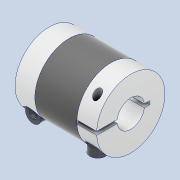
# Autodesk Inventor part: Coupling_SOH-16C-5×6_自作モデル
Saved by Autodesk Inventor 2021.2 (Build 252289000, 289)
## iProperties
Created: 2021-02-28
Part Number: Coupling_SOH-16C-5×6_自作モデル
Material: アルミニウム 6061
Document SubType Name: Modeling
Designer: Hagihara Yuya
Density: 2.7 g/cm^3
Appearance: アルミニウム - フラット
Author: Hagihara Yuya
Autodesk Inventor part; units mm, degrees
sketch "スケッチ1" plane through (0, 0, 0) normal (1, 0, 0) x (0, 1, 0)
  circle A0 centre (0, 0) radius 10
  dimension "d0" = 20
  constraints: 1 centre point, 1 coincident
  measures "d0" diameter of A0
extrude "押し出し1" add sketch "スケッチ1" along normal blind 23.9
sketch "スケッチ2" plane through (23.9, 0, 0) normal (1, 0, 0) x (0, 0, -1)
  point P0 (0, 0)
  point P1 (0, 0)
  constraints: 1 coincident
hole "軸穴1" at (23.9, 0, 0) direction (-1, 0, 0) diameter 8 depth 11
sketch "スケッチ3" plane through (0, 0, 0) normal (-1, 0, 0) x (0, 0, 1)
  point P0 (0, 0)
  point P1 (0, 0)
  constraints: 1 coincident
hole "軸穴2" at (0, 0, 0) direction (1, 0, 0) diameter 8 depth 11
ref_plane "作業平面1" through (5.8, 0, 0) normal (-1, 0, 0) x (0, 0, 1)
sketch "スケッチ4" plane through (5.8, 0, 0) normal (-1, 0, 0) x (0, 0, 1)
  circle A0 centre (0, 0) radius 9.99
  circle A1 centre (0, 0) radius 10 projected
  dimension "d18" = 0.01
  constraints: 1 centre point, 1 coincident
  measures "d18" radial gap between concentric circles of A1 A0
extrude "押し出し2" cut sketch "スケッチ4" against normal blind 12.3
sketch "スケッチ5" plane through (23.9, 0, 0) normal (1, 0, 0) x (0, 0, -1)
  line L0 (-5.5, -0.5) -> (10, -0.5)
  line L1 (10, -0.5) -> (10, 0.5)
  line L2 (10, 0.5) -> (-5.5, 0.5)
  line L3 (-5.5, 0.5) -> (-5.5, -0.5)
  circle A0 centre (0, 0) radius 10 projected
  point P0 (-5.5, 0)
  point P1 (9.9875, -0.5)
  point P2 (9.9875, 0.5)
  dimension "d21" = 1
  dimension "d22" = 5.5
  constraints: 8 end point, 2 parallel, 1 horizontal, 1 horizontal alignment, 1 midpoint, 1 perpendicular, 1 tangent
  measures "d21" distance of L2.end L0.start
  measures "d22" distance from line of point (0, 0) L3
extrude "スリット1" cut sketch "スケッチ5" against normal up to surface (5.8 mm away) contours L3 L2 A0 L0 picked at (-0.3333, 0)
sketch "スケッチ6" plane through (0, 0, 0) normal (-1, 0, 0) x (0, 0, 1)
  line L0 (-0.5, 10) -> (0.5, 10)
  line L1 (0.5, 10) -> (0.5, -5.5)
  line L2 (0.5, -5.5) -> (-0.5, -5.5)
  line L3 (-0.5, -5.5) -> (-0.5, 10)
  circle A0 centre (0, 0) radius 10 projected
  point P0 (0, -5.5)
  dimension "d25" = 1
  dimension "d26" = 5.5
  constraints: 8 end point, 2 parallel, 1 horizontal, 1 midpoint, 1 perpendicular, 1 tangent, 1 vertical alignment
  measures "d25" distance of L1.end L2.end
  measures "d26" distance from line of L2 point (0, 0)
extrude "スリット2" cut sketch "スケッチ6" against normal up to surface (5.8 mm away) contours L0 A0 L3 | L0 L1 A0 | A0 L1 L2 L3 picked at (0, -0.3333)
ref_plane "作業平面2" through (23.9, 10, -9.9875) normal (0, -1, 0) x (1, 0, 0)
sketch "スケッチ7" plane through (23.9, 10, -9.9875) normal (0, -1, 0) x (1, 0, 0)
  line L0 (0, 0) -> (0, 19.9875) projected
  point P0 (-23.9, 9.9875)
  point P1 (-2.9, 2.9875)
  dimension "d30" = 2.9
  dimension "d68" = 7
  measures "d30" distance from line of L0 point (-2.9, 2.987)
  measures "d68" vertical distance of point (-23.9, 9.987) point (-2.9, 2.987)
hole "ボルト穴1" at (21, 10, -7) direction (0, -1, 0) diameter 2.1129 end through all counterbore diameter 5 counterbore depth 5 thread size "M2.6x0.45" class "6H" standard "ISO Metric profile"
ref_plane "作業平面3" through (0, 3.9686, -10) normal (0, 0, 1) x (1, 0, 0)
sketch "スケッチ8" plane through (0, 3.9686, -10) normal (0, 0, 1) x (1, 0, 0)
  line L0 (0, -13.9686) -> (0, 6.0189) projected
  point P0 (0, -3.9686)
  point P1 (2.7, 3.0314)
  dimension "d40" = 2.7
  dimension "d41" = 7
  measures "d40" distance from line of L0 point (2.7, 3.031)
  measures "d41" vertical distance of point (2.7, 3.031) point (0, -3.969)
hole "ボルト穴2" at (2.7, 7, -10) direction (0, 0, 1) diameter 2.1129 end through all counterbore diameter 5 counterbore depth 5 thread size "M2.6x0.45" class "6H" standard "ISO Metric profile"
sketch "スケッチ12" plane through (21, 5, -7) normal (0, 1, 0) x (1, 0, 0)
  circle A0 centre (0, 0) radius 1.0564 projected
  circle A1 centre (0, 0) radius 2.25
  point P0 (-21, -7)
  dimension "d60" = 4.5
  constraints: 1 centre point, 1 coincident
  measures "d60" diameter of A1
extrude "ネジ頭1" add sketch "スケッチ12" along normal blind 2.6 separate body contours A0 | A1
sketch "スケッチ13" plane through (21, 5, -7) normal (0, -1, 0) x (1, 0, 0)
  circle A0 centre (0, 0) radius 2.25 projected
  circle A1 centre (0, 0) radius 1.3
  circle A2 centre (0, 0) radius 1.0564 projected
  point P0 (-21, 7)
  dimension "d63" = 2.6
  constraints: 1 centre point, 1 coincident
  measures "d63" diameter of A1
extrude "ネジ1" add sketch "スケッチ13" along normal blind 8 separate body contours A2
thread "ねじ1" size "M2.2x0.45" class "6g" standard "ISO Metric profile" full length
sketch "スケッチ14" plane through (21, 7.6, -7) normal (0, 1, 0) x (1, 0, 0)
  circle A0 centre (0, 0) radius 2.25 projected
  line L0 (1, -0.5774) -> (0, -1.1547)
  line L1 (0, -1.1547) -> (-1, -0.5774)
  line L2 (-1, -0.5774) -> (-1, 0.5774)
  line L3 (-1, 0.5774) -> (0, 1.1547)
  line L4 (0, 1.1547) -> (1, 0.5774)
  line L5 (1, 0.5774) -> (1, -0.5774)
  point P0 (-21, -7)
  dimension "d69" = 2
  constraints: 12 end point, 1 coincident, 1 vertical alignment, 13 other
  measures "d69" distance between parallel lines of L2 L5
extrude "六角穴1" cut sketch "スケッチ14" against normal blind 1.1 contours L0 L1 L2 L3 L4 L5 bodies 2
sketch "スケッチ9" plane through (2.7, 7, -5) normal (0, 0, -1) x (-1, 0, 0)
  circle A0 centre (0, 0) radius 1.0564 projected
  circle A1 centre (0, 0) radius 2.25
  point P0 (2.7, -7)
  dimension "d49" = 4.5
  constraints: 1 centre point, 1 coincident
  measures "d49" diameter of A1
extrude "ネジ頭2" add sketch "スケッチ9" along normal blind 2.6 separate body contours A0 | A1
sketch "スケッチ10" plane through (2.7, 7, -5) normal (0, 0, 1) x (1, 0, 0)
  circle A0 centre (0, 0) radius 1.0564 projected
  circle A1 centre (0, 0) radius 1.3
  point P0 (-2.7, -7)
  dimension "d52" = 2.6
  constraints: 1 centre point, 1 coincident
  measures "d52" diameter of A1
extrude "ネジ2" add sketch "スケッチ10" along normal blind 8 separate body contours A0
thread "ねじ2" size "M2.6x0.45" class "6g" standard "ISO Metric profile" full length
sketch "スケッチ11" plane through (2.7, 7, -7.6) normal (0, 0, -1) x (-1, 0, 0)
  line L0 (-0.5774, -1) -> (-1.1547, 0)
  line L1 (-1.1547, 0) -> (-0.5774, 1)
  line L2 (-0.5774, 1) -> (0.5774, 1)
  line L3 (0.5774, 1) -> (1.1547, 0)
  line L4 (1.1547, 0) -> (0.5774, -1)
  line L5 (0.5774, -1) -> (-0.5774, -1)
  point P0 (2.7, -7)
  point P1 (0, 0)
  point P2 (0, 0)
  dimension "d57" = 2
  constraints: 12 end point, 1 coincident, 1 horizontal alignment, 13 other
  measures "d57" distance between parallel lines of L2 L5
extrude "六角穴2" cut sketch "スケッチ11" against normal blind 1.1 bodies 4
equation "\"d0\" = 外径"
equation "\"d3\" = 軸穴径1"
equation "\"d10\" = 軸穴径2"
equation "\"d19\" = d1 + 2 * d17"
equation "\"d23\" = d1 + 2 * d17"
equation "\"d27\" = d1 + 2 * d17"
equation "\"d30\" = ボルト位置"
equation "\"d68\" = 0.25 * 軸穴径1 + 0.25 * 外径"
equation "\"d41\" = 0.25 * 軸穴径2 + 0.25 * 外径"
equation "\"d17\" = -2 * ボルト位置"
equation "\"d31\" = 0.25 * d10 + 0.25 * d0"
equation "\"軸穴径1\" = 8"
equation "\"軸穴径2\" = 8"
equation "\"外径\" = 20"
equation "\"全長\" = 21.9"
equation "\"ボルト位置\" = 2.9"
equation "\"d1\" = 23.9"
